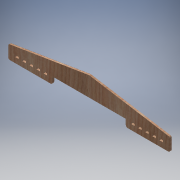
# Autodesk Inventor part: TrusSupport
Saved by Autodesk Inventor 2019 (Build 230136000, 136)
## iProperties
Created: 2019-01-19
Part Number: TrusSupport
Material: Wood (Birch)
Document SubType Name: Modeling
Designer: nxgam
Density: 0.55 g/cm^3
Appearance: Birch - Natural Polished
Author: nxgam
Autodesk Inventor part; units mm, degrees
ref_plane "YZ Plane" through (0, 0, 0) normal (1, 0, 0) x (0, 1, 0)
ref_plane "XZ Plane" through (0, 0, 0) normal (0, 1, 0) x (-1, 0, 0)
ref_plane "XY Plane" through (0, 0, 0) normal (0, 0, 1) x (1, 0, 0)
sketch "Sketch1" plane through (0, 0, 0) normal (0, 0, 1) x (1, 0, 0)
  line L0 (-232.2957, 0) -> (232.2957, 0)
  line L1 (232.2957, 0) -> (232.2957, 38.1)
  line L2 (232.2957, 38.1) -> (-232.2957, 38.1) construction
  line L3 (-232.2957, 38.1) -> (-232.2957, 0)
  line L4 (-232.2957, 38.1) -> (0, 76.2)
  line L5 (0, 76.2) -> (232.2957, 38.1)
  line L6 (0, 76.2) -> (0, 38.1) construction
  point P0 (0, 0)
  point P1 (0, 0)
  dimension "d0" = 464.5914
  dimension "d1" = 38.1
  dimension "d2" = 38.1
  constraints: 14 end point, 2 midpoint, 2 parallel, 2 perpendicular, 1 coincident, 1 horizontal
  measures "d0" distance of L2.end L1.end
  measures "d1" distance of L0.end L1.end
  measures "d2" distance of L4.end L6.end
extrude "Extrusion1" add sketch "Sketch1" along normal blind 5.08
fillet "Fillet1" radius 5.08 3 edges at (0, 76.2, 2.54) (232.2957, 38.1, 2.54) (-232.2957, 38.1, 2.54)
fillet "Fillet2" radius 5.08 2 edges at (-232.2957, 0, 2.54) (232.2957, 0, 2.54)
sketch "Sketch2" plane through (0, 0, 0) normal (0, 0, -1) x (-1, 0, 0)
  line L0 (-211.9778, 20.32) -> (-201.8178, 20.32)
  line L1 (-201.8178, 20.32) -> (-201.8178, 15.24)
  line L2 (-201.8178, 15.24) -> (-211.9778, 15.24)
  line L3 (-211.9778, 15.24) -> (-211.9778, 20.32)
  line L4 (-191.6578, 20.32) -> (-181.4978, 20.32)
  line L5 (-181.4978, 20.32) -> (-181.4978, 15.24)
  line L6 (-181.4978, 15.24) -> (-191.6578, 15.24)
  line L7 (-191.6578, 15.24) -> (-191.6578, 20.32)
  line L8 (-171.3378, 20.32) -> (-161.1778, 20.32)
  line L9 (-161.1778, 20.32) -> (-161.1778, 15.24)
  line L10 (-161.1778, 15.24) -> (-171.3378, 15.24)
  line L11 (-171.3378, 15.24) -> (-171.3378, 20.32)
  line L12 (-151.0178, 20.32) -> (-140.8578, 20.32)
  line L13 (-140.8578, 20.32) -> (-140.8578, 15.24)
  line L14 (-140.8578, 15.24) -> (-151.0178, 15.24)
  line L15 (-151.0178, 15.24) -> (-151.0178, 20.32)
  line L16 (-130.6978, 20.32) -> (-120.5378, 20.32)
  line L17 (-120.5378, 20.32) -> (-120.5378, 15.24)
  line L18 (-120.5378, 15.24) -> (-130.6978, 15.24)
  line L19 (-130.6978, 15.24) -> (-130.6978, 20.32)
  line L20 (-45.72, 20.32) -> (-45.72, 15.24)
  line L21 (-45.72, 15.24) -> (-105.2978, 15.24) construction
  line L22 (-105.2978, 15.24) -> (-105.2978, 20.32)
  line L23 (-105.2978, 20.32) -> (-45.72, 20.32)
  line L24 (-40.64, 15.24) -> (-40.64, 20.32)
  line L25 (-40.64, 20.32) -> (40.64, 20.32)
  line L26 (40.64, 20.32) -> (40.64, 15.24)
  line L27 (40.64, 15.24) -> (-40.64, 15.24) construction
  line L28 (45.72, 15.24) -> (45.72, 20.32)
  line L29 (45.72, 20.32) -> (105.2978, 20.32)
  line L30 (105.2978, 20.32) -> (105.2978, 15.24)
  line L31 (105.2978, 15.24) -> (45.72, 15.24) construction
  arc A0 (-232.2957, 5.08) -> (-227.2157, 0) centre (-227.2157, 5.08) ccw projected
  line L32 (227.2157, 0) -> (-227.2157, 0) projected
  arc A1 (227.2157, 0) -> (232.2957, 5.08) centre (227.2157, 5.08) ccw projected
  line L33 (232.2957, 33.7853) -> (232.2957, 5.08) projected
  arc A2 (232.2957, 33.7853) -> (228.0379, 38.7983) centre (227.2157, 33.7853) ccw projected
  line L34 (0.8222, 76.0651) -> (228.0379, 38.7983) construction
  arc A3 (0.8222, 76.0651) -> (-0.8222, 76.0651) centre (0, 71.0521) ccw construction
  line L35 (-228.0379, 38.7983) -> (-0.8222, 76.0651) construction
  arc A4 (-228.0379, 38.7983) -> (-232.2957, 33.7853) centre (-227.2157, 33.7853) ccw projected
  line L36 (-232.2957, 5.08) -> (-232.2957, 33.7853) projected
  line L37 (-105.2978, 15.24) -> (-105.2978, 0)
  line L38 (227.2157, 0) -> (-227.2157, 0) projected
  line L39 (-105.2978, 20.32) -> (105.2978, 20.32)
  line L40 (105.2978, 20.32) -> (105.2978, 0)
  line L41 (105.2978, 0) -> (-105.2978, 0)
  line L42 (-105.2978, 0) -> (-105.2978, 20.32)
  point P0 (0, 0)
  constraints: 74 end point, 17 horizontal, 16 vertical, 2 parallel, 2 perpendicular, 2 point on line, 32 other
extrude "Extrusion2" cut sketch "Sketch2" against normal blind 5.08
fillet "Fillet3" radius 5.08 2 edges at (105.2978, 0, 2.54) (-105.2978, 0, 2.54)
mirror "Mirror1" about plane through (0, 0, 0) normal (1, 0, 0) of "Extrusion2"
body "Solid1"
